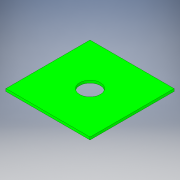
# Autodesk Inventor part: Base_tapa
Saved by Autodesk Inventor 2019 (Build 230136000, 136)
## iProperties
Created: 2020-02-05
Part Number: Base_tapa
Material: Generic
Document SubType Name: Modeling
Designer: Omar
Density: 1 g/cm^3
Appearance: Default
Author: Omar
Autodesk Inventor part; units mm, degrees
ref_plane "YZ Plane" through (0, 0, 0) normal (1, 0, 0) x (0, 1, 0)
ref_plane "XZ Plane" through (0, 0, 0) normal (0, 1, 0) x (-1, 0, 0)
ref_plane "XY Plane" through (0, 0, 0) normal (0, 0, 1) x (1, 0, 0)
sketch "Sketch1" plane through (0, 0, 0) normal (0, 1, 0) x (-1, 0, 0)
  line L0 (-53.18, 53.18) -> (53.18, 53.18)
  line L1 (53.18, 53.18) -> (53.18, -53.18)
  line L2 (53.18, -53.18) -> (-53.18, -53.18)
  line L3 (-53.18, -53.18) -> (-53.18, 53.18)
  line L4 (-53.18, 53.18) -> (53.18, -53.18) construction
  line L5 (53.18, 53.18) -> (-53.18, -53.18) construction
  circle A0 centre (0, 0) radius 13
  dimension "d0" = 106.36
  dimension "d1" = 106.36
  dimension "d2" = 26
  constraints: 12 end point, 2 midpoint, 2 parallel, 1 centre point, 1 coincident, 1 horizontal, 1 perpendicular
  measures "d0" distance of L1.end L2.end
  measures "d1" distance of L0.end L1.end
  measures "d2" diameter of A0
extrude "Extrusion1" add sketch "Sketch1" along normal blind 3.18
body "Solid1"
